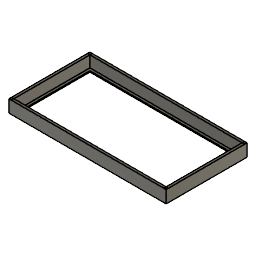
front_frame (Autodesk Fusion 360 design; units mm, degrees)
part number: 2026-05-14-23-54-17-745
Autodesk Fusion 360 part; units mm, degrees
sketch "Sketch1" plane through (0, 0, 0) normal (0, 0, 1) x (1, 0, 0)
  line L0 (-51.0433, -16.8971) -> (557.9567, -16.8971)
  line L1 (557.9567, -16.8971) -> (557.9567, 287.1029)
  line L2 (557.9567, 287.1029) -> (-51.0433, 287.1029)
  line L3 (-51.0433, 287.1029) -> (-51.0433, -16.8971)
  line L4 (-41.0433, -6.8971) -> (547.9567, -6.8971)
  line L5 (547.9567, -6.8971) -> (547.9567, 277.1029)
  line L6 (547.9567, 277.1029) -> (-41.0433, 277.1029)
  line L7 (-41.0433, 277.1029) -> (-41.0433, -6.8971)
  line L8 (-61.0433, -26.8971) -> (567.9567, -26.8971)
  line L9 (567.9567, -26.8971) -> (567.9567, 297.1029)
  line L10 (567.9567, 297.1029) -> (-61.0433, 297.1029)
  line L11 (-61.0433, 297.1029) -> (-61.0433, -26.8971)
  circle A0 centre (-55.5433, -21.3971) radius 5
  circle A1 centre (-55.5433, 291.6029) radius 5
  circle A2 centre (562.4567, 291.6029) radius 5
  circle A3 centre (562.4567, -21.3971) radius 5
  dimension "d1" = 609
  dimension "d2" = 304
  dimension "d3" = 10
  dimension "d4" = 10
  dimension "d5" = 10
  dimension "d6" = 10
  dimension "d7" = 10
  dimension "d8" = 10
  dimension "d9" = 10
  dimension "d10" = 10
  dimension "d11" = 10
  dimension "d12" = 5.5
  dimension "d13" = 5.5
  dimension "d14" = 10
  dimension "d15" = 5.5
  dimension "d16" = 5.5
  dimension "d17" = 10
  dimension "d18" = 5.5
  dimension "d19" = 5.5
  dimension "d20" = 10
  dimension "d21" = 5.5
  dimension "d22" = 5.5
  constraint horizontal L0
  constraint vertical L1
  constraint horizontal L2
  constraint vertical L3
  constraint horizontal L4
  constraint vertical L5
  constraint horizontal L6
  constraint vertical L7
  constraint horizontal L8
  constraint vertical L9
  constraint horizontal L10
  constraint vertical L11
  measures "d1" distance of L0.start L0.end
  measures "d2" distance of L0.start L2.end
  measures "d3" distance of L2 L6
  measures "d4" distance of L0 L4
  measures "d5" distance of L3 L7
  measures "d6" distance of L1 L5
  measures "d7" distance of L2 L10
  measures "d8" distance of L1 L9
  measures "d9" distance of L0 L8
  measures "d10" distance of L3 L11
  measures "d11" diameter of A0
  measures "d12" distance of L8 A0.centre
  measures "d13" distance of L11 A0.centre
  measures "d14" diameter of A1
  measures "d15" distance of L10 A1.centre
  measures "d16" distance of L11 A1.centre
  measures "d17" diameter of A2
  measures "d18" distance of L10 A2.centre
  measures "d19" distance of L9 A2.centre
  measures "d20" diameter of A3
  measures "d21" distance of L9 A3.centre
  measures "d22" distance of L8 A3.centre
extrude "Extrude1" add sketch "Sketch1" along normal blind 5 contours L0 L1 L2 L3
extrude "Extrude2" add sketch "Sketch1" along normal blind 50 contours L8 L9 L10 L11
